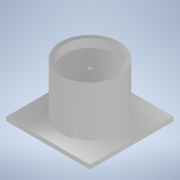
# Autodesk Inventor part: C0
Saved by Autodesk Inventor 2022.2 (Build 262287010, 287A)
## iProperties
Created: 2022-04-10
Part Number: C0
Material: Aluminum 6061
Document SubType Name: Modeling
Designer: stasi
Density: 2.7 g/cm^3
Appearance: Aluminum - Flat
Mass: 2704.36 g
Surface Area: 1827.19 cm^2
Volume: 1001.61 cm^3
Author: stasi
Autodesk Inventor part; units mm, degrees
ref_plane "YZ Plane" through (0, 0, 0) normal (1, 0, 0) x (0, 1, 0)
ref_plane "XZ Plane" through (0, 0, 0) normal (0, 1, 0) x (-1, 0, 0)
ref_plane "XY Plane" through (0, 0, 0) normal (0, 0, 1) x (1, 0, 0)
sketch "Sketch1" plane through (0, 0, 0) normal (0, 1, 0) x (-1, 0, 0)
  line L0 (-100, 100) -> (100, 100)
  line L1 (100, 100) -> (100, -100)
  line L2 (100, -100) -> (-100, -100)
  line L3 (-100, -100) -> (-100, 100)
  line L4 (-100, 100) -> (100, -100) construction
  line L5 (100, 100) -> (-100, -100) construction
  point P0 (0, 0)
  dimension "d0" = 200
  dimension "d1" = 200
  constraints: 12 end point, 2 midpoint, 2 parallel, 1 horizontal, 1 perpendicular
  measures "d0" distance of L1.end L2.end
  measures "d1" distance of L0.end L1.end
extrude "podstawa na mocowanie" add sketch "Sketch1" along normal blind 10
sketch "Sketch2" plane through (0, 10, 0) normal (0, 1, 0) x (1, 0, 0)
  circle A0 centre (0, 0) radius 70
  circle A1 centre (0, 0) radius 60
  dimension "d4" = 140
  dimension "d5" = 120
  constraints: 2 centre point, 2 coincident
  measures "d4" diameter of A0
  measures "d5" diameter of A1
extrude "trzon c0" add sketch "Sketch2" along normal blind 120
sketch "Sketch5" plane through (0, 10, 0) normal (0, 1, 0) x (1, 0, 0)
  circle A0 centre (0, 0) radius 60 projected
  circle A1 centre (0, 0) radius 60
  dimension "d19" = 120
  constraints: 1 centre point, 1 coincident
  measures "d19" diameter of A1
extrude "wneka na silnik c0" cut sketch "Sketch5" against normal blind 10
sketch "Sketch6" plane through (0, 130, 0) normal (0, 1, 0) x (1, 0, 0)
  circle A0 centre (0, 0) radius 60
  dimension "d20" = 120
  constraints: 1 centre point, 1 coincident
  measures "d20" diameter of A0
extrude "powierzchnia nosna dla c1" add sketch "Sketch6" against normal blind 40
sketch "Sketch8" plane through (0, 130, 0) normal (0, 1, 0) x (1, 0, 0)
  circle A0 centre (0, 0) radius 60
  dimension "d13" = 120
  constraints: 1 centre point, 1 coincident
  measures "d13" diameter of A0
extrude "wneka na podstawe c1" cut sketch "Sketch8" against normal blind 20
sketch "Sketch9" plane through (0, 110, 0) normal (0, 1, 0) x (1, 0, 0)
  circle A0 centre (0, 0) radius 5
  dimension "d16" = 10
  constraints: 1 centre point, 1 coincident
  measures "d16" diameter of A0
extrude "dziura na wal c1" cut sketch "Sketch9" against normal blind 20
body "Solid1"
